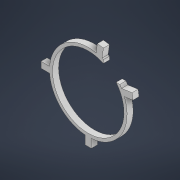
# Autodesk Inventor part: Clip_TestFitV1
Saved by Autodesk Inventor 2022 (Build 260153000, 153)
## iProperties
Created: 2023-05-05
Part Number: Clip_TestFitV1
Material: Generic
Document SubType Name: Modeling
Designer: User
Density: 1 g/cm^3
Appearance: Default
Author: User
Autodesk Inventor part; units mm, degrees
ref_plane "YZ Plane" through (0, 0, 0) normal (1, 0, 0) x (0, 1, 0)
ref_plane "XZ Plane" through (0, 0, 0) normal (0, 1, 0) x (-1, 0, 0)
ref_plane "XY Plane" through (0, 0, 0) normal (0, 0, 1) x (1, 0, 0)
sketch "Sketch1" plane through (0, 0, 0) normal (0, 0, 1) x (1, 0, 0)
  arc A0 (-25.4018, 15) -> (25.4018, 15) centre (0, 0) ccw
  line L0 (-39, 2.5) -> (-32, 2.5)
  line L1 (-32, -2.5) -> (-39, -2.5)
  line L2 (-39, -2.5) -> (-39, 2.5)
  line L3 (-32, 2.5) -> (-31.9022, 2.5)
  line L4 (-32, -2.5) -> (-31.9022, -2.5)
  line L5 (2.5, -32) -> (2.5, -39)
  line L6 (2.5, -39) -> (-2.5, -39)
  line L7 (-2.5, -39) -> (-2.5, -32)
  line L8 (-2.5, -32) -> (-2.5, -31.9022)
  line L9 (2.5, -32) -> (2.5, -31.9022)
  line L10 (32, 2.5) -> (31.9022, 2.5)
  line L11 (32, -2.5) -> (31.9022, -2.5)
  arc A1 (-28.2666, 15) -> (-31.9022, 2.5) centre (0, 0) ccw
  arc A2 (-31.9022, -2.5) -> (-2.5, -31.9022) centre (0, 0) ccw
  arc A3 (2.5, -31.9022) -> (31.9022, -2.5) centre (0, 0) ccw
  arc A4 (31.9022, 2.5) -> (28.2666, 15) centre (0, 0) ccw
  arc A5 (12.5, 26.7208) -> (25.4018, 15) centre (0, 0) ccw
  line L12 (12.5, 29.4576) -> (12.5, 26.7208)
  arc A6 (-2.5, 31.9022) -> (-31.9022, 2.5) centre (0, 0) ccw
  arc A7 (-31.9022, -2.5) -> (-2.5, -31.9022) centre (0, 0) ccw
  arc A8 (2.5, -31.9022) -> (31.9022, -2.5) centre (0, 0) ccw
  arc A9 (31.9022, 2.5) -> (28.2666, 15) centre (0, 0) ccw
  line L13 (6.5, 31.3329) -> (7.5001, 38.3601)
  line L14 (6.5, 31.3329) -> (13.598, 31.3329) construction
  line L15 (7.5001, 38.3601) -> (12.4502, 37.6556)
  line L16 (12.4502, 37.6556) -> (11.3493, 29.9198)
  arc A10 (12.5, 29.4576) -> (11.3493, 29.9198) centre (0, 0) ccw
  arc A11 (12.5, 29.4576) -> (11.3493, 29.9198) centre (0, 0) ccw
  arc A12 (6.5, 31.3329) -> (2.5, 31.9022) centre (0, 0) ccw
  arc A13 (6.5, 31.3329) -> (-31.9022, 2.5) centre (0, 0) ccw
  arc A14 (31.9022, 2.5) -> (28.2666, 15) centre (0, 0) ccw
  arc A15 (-31.9022, -2.5) -> (-2.5, -31.9022) centre (0, 0) ccw
  arc A16 (2.5, -31.9022) -> (31.9022, -2.5) centre (0, 0) ccw
  line L17 (31.9022, 2.5) -> (41.0332, 2.5) construction
  line L18 (29.8114, 11.631) -> (36.8386, 12.6311)
  line L19 (29.8114, 11.631) -> (36.9094, 11.631) construction
  line L20 (36.8386, 12.6311) -> (41.8386, 12.6311) construction
  line L21 (36.8386, 12.6311) -> (36.1341, 17.5812)
  line L22 (36.8386, 12.6311) -> (41.8386, 12.6311) construction
  line L23 (36.1341, 17.5812) -> (27.5058, 16.3533)
  line L24 (36.1341, 17.5812) -> (44.8493, 17.5812) construction
  arc A17 (12.5, 26.7208) -> (24.5524, 16.3533) centre (0, 0) ccw
  arc A18 (12.5, 29.4576) -> (11.3493, 29.9198) centre (0, 0) ccw
  arc A19 (2.5, -31.9022) -> (27.5058, 16.3533) centre (0, 0) ccw
  arc A20 (6.5, 31.3329) -> (-31.9022, 2.5) centre (0, 0) ccw
  arc A21 (-31.9022, -2.5) -> (-2.5, -31.9022) centre (0, 0) ccw
  arc A22 (12.5, 26.7208) -> (22.9783, 18.5) centre (0, 0) ccw
  line L25 (28.2666, 15) -> (31.7666, 15) construction
  line L26 (22.9783, 18.5) -> (26.1103, 18.5)
  arc A23 (12.5, 29.4576) -> (11.3493, 29.9198) centre (0, 0) ccw
  arc A24 (6.5, 31.3329) -> (-31.9022, 2.5) centre (0, 0) ccw
  arc A25 (-31.9022, -2.5) -> (-2.5, -31.9022) centre (0, 0) ccw
  arc A26 (2.5, -31.9022) -> (26.1103, 18.5) centre (0, 0) ccw
  point P0 (11.5, 29.8622)
  point P1 (2.5, 31.9022)
  point P2 (24.5524, 16.3533)
  point P3 (25.4018, 15)
  dimension "d78" = 7.098
  dimension "d79" = 81.9
  dimension "d80" = 5
  dimension "d81" = 90
  dimension "d82" = 90
  dimension "d89" = 7.098
  dimension "d90" = 8.1
  dimension "d93" = 5
  dimension "d94" = 98.1
  dimension "d95" = 171.9
  constraints: 55 point on circle, 54 end point, 27 centre point, 13 horizontal, 9 coincident, 4 equal length, 2 concentric, 2 parallel, 2 vertical, 1 perpendicular
  measures "d78" distance of L13.start L13.end
  measures "d79" angle of L14 L13
  measures "d80" distance of L13.end L15.end
  measures "d81" angle of L13 L15
  measures "d82" angle of L15 L16
  measures "d89" distance of L18.start L18.end
  measures "d90" angle of L19 L18
  measures "d93" distance of L18.end L21.end
  measures "d94" angle of L22 L21
  measures "d95" angle of L23 L24
extrude "Extrusion7" add sketch "Sketch1" along normal blind 5
body "Solid5"
